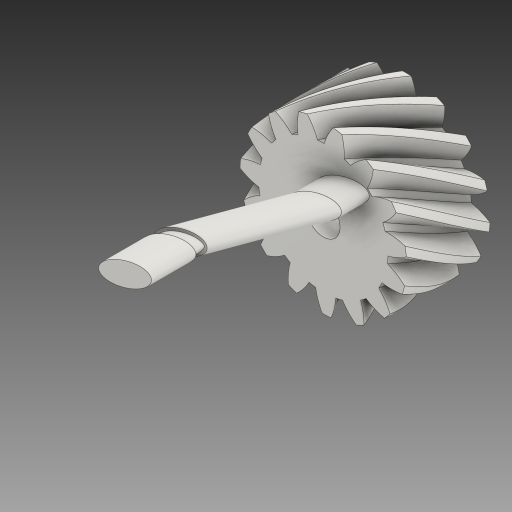
# Autodesk Inventor part: Finger_Profil_V2
Saved by Autodesk Inventor 2024 (Build 280153000, 153)
## iProperties
CustomPartVersion: 1
Created: 2024-03-13
Part Number: Finger_Profil_V2
Material: Steel
Document SubType Name: Modeling
Designer: Faber
Categories: <?xml version="1.0" encoding="UTF-16"?> <MemberInstance><Categories><FamilyTemplate><FamilyTemplateParameter ValueType="xs:double" Id="1" ObjectReferenceKey="da_z" ObjectType="kUserParameterObject"/><FamilyTemplateParameter ValueType="xs:double" Id="2" ObjectReferenceKey="da_b" ObjectType="kUserParameterObject"/><FamilyTemplateParameter ValueType="xs:double" Id="3" ObjectReferenceKey="da_beta" ObjectType="kUserParameterObject"/><FamilyTemplateParameter ValueType="xs:double" Id="4" ObjectReferenceKey="da_da" ObjectType="kUserParameterObject"/><FamilyTemplateParameter ValueType="xs:double" Id="5" ObjectReferenceKey="da_aw" ObjectType="kUserParameterObject"/><FamilyTemplateParameter ValueType="xs:string" Id="6" ObjectReferenceKey="EAIAABAAAACIAQAAAAAAAIAAAAAAAAAA" ObjectType="83910656" SubObjectId="SurfaceGeometry"/></FamilyTemplate><ParamToTemplateMap><ParamToTemplate CategoryParameter="//CategoryParameter[@InternalName='046C89C9-8512-4d59-83FE-43B91F4F132A']" TemplateParameter="1"/><ParamToTemplate CategoryParameter="//CategoryParameter[@InternalName='2552DF32-E462-4b46-AEBF-C6C7768E72AC']" TemplateParameter="2"/><ParamToTemplate CategoryParameter="//CategoryParameter[@InternalName='C9EE641D-15FC-4fae-A226-E94C4372FDD7']" TemplateParameter="3"/><ParamToTemplate><ParamToTemplate CategoryParameter="//CategoryParameter[@InternalName='00B6519A-459B-49c7-AD84-2E56D39A5744']" ConstantValue="0.340699"/></ParamToTemplate><ParamToTemplate><ParamToTemplate CategoryParameter="//CategoryParameter[@InternalName='04B31F0E-C7A6-4894-AA32-9629BEFACF47']" ConstantValue="1.000000"/></ParamToTemplate><ParamToTemplate><ParamToTemplate CategoryParameter="//CategoryParameter[@InternalName='43CBEC2E-7847-49e7-A936-2F7889FCB2D9']" ConstantValue="0.250000"/></ParamToTemplate><ParamToTemplate><ParamToTemplate CategoryParameter="//CategoryParameter[@InternalName='B1EFC894-105D-4ebd-86BF-FA20ED196853']" ConstantValue="0.333500"/></ParamToTemplate><ParamToTemplate><ParamToTemplate CategoryParameter="//CategoryParameter[@InternalName='51175063-3D10-4879-93E8-6246FE8B403D']" ConstantValue="2060000000.000000"/></ParamToTemplate><ParamToTemplate><ParamToTemplate CategoryParameter="//CategoryParameter[@InternalName='A3A52E27-4454-46a9-B0BD-C932399B70AF']" ConstantValue="0.300000"/></ParamToTemplate><ParamToTemplate><ParamToTemplate CategoryParameter="//CategoryParameter[@InternalName='91B76062-C214-41d9-B1B9-14D2AB99603D']" ConstantValue="0.150000"/></ParamToTemplate><ParamToTemplate><ParamToTemplate CategoryParameter="//CategoryParameter[@InternalName='374E806E-8B8A-4dda-A9AA-1039D6500AD2']" ConstantValue="6.666667"/></ParamToTemplate><ParamToTemplate><ParamToTemplate CategoryParameter="//CategoryParameter[@InternalName='2D373A89-B862-43d6-8D0B-0CBF12AB9F6C']" ConstantValue="0.349066"/></ParamToTemplate><ParamToTemplate CategoryParameter="//CategoryParameter[@InternalName='37777632-D6A2-4fac-9D53-DB8ACD95C989']" TemplateParameter="4"/><ParamToTemplate CategoryParameter="//CategoryParameter[@InternalName='FD1017F1-B727-4f7e-9707-0F86F1FF9423']" TemplateParameter="5"/><ParamToTemplate><ParamToTemplate CategoryParameter="//CategoryParameter[@InternalName='9E1B4470-B2D3-4ff1-B813-535BB4CDF51A']" ConstantValue="3520000.000000"/></ParamToTemplate><ParamToTemplate><ParamToTemplate CategoryParameter="//CategoryParameter[@InternalName='F8452263-BFF6-458c-9FB1-07C4B99E95CD']" ConstantValue="11400000.000000"/></ParamToTemplate><ParamToTemplate><ParamToTemplate CategoryParameter="//CategoryParameter[@InternalName='3E3BB259-FD49-497f-8171-6EBC954A3479']" ConstantValue="2.000000"/></ParamToTemplate><ParamToTemplate CategoryParameter="//CategoryParameter[@InternalName='27C3BAF2-7550-4e4b-AE2C-0DB134B7D9B7']" TemplateParameter="6"/></ParamToTemplateMap><Category DisplayName="Gear" InternalName="DC85795E-93AB-48d5-8EEE-5A27447B64BD" Mnemonic="Gear"><CategoryParameter DisplayName="z" InternalName="046C89C9-8512-4d59-83FE-43B91F4F132A" Mnemonic="z"/><CategoryParameter DisplayName="b" InternalName="2552DF32-E462-4b46-AEBF-C6C7768E72AC" Mnemonic="b"/><CategoryParameter DisplayName="||b|" InternalName="C9EE641D-15FC-4fae-A226-E94C4372FDD7" Mnemonic="beta"/><CategoryParameter DisplayName="x" InternalName="00B6519A-459B-49c7-AD84-2E56D39A5744" Mnemonic="x"/><CategoryParameter DisplayName="a*" InternalName="04B31F0E-C7A6-4894-AA32-9629BEFACF47" Mnemonic="a"/><CategoryParameter DisplayName="c*" InternalName="43CBEC2E-7847-49e7-A936-2F7889FCB2D9" Mnemonic="c"/><CategoryParameter DisplayName="r|.f|*" InternalName="B1EFC894-105D-4ebd-86BF-FA20ED196853" Mnemonic="rf"/><CategoryParameter DisplayName="E" InternalName="51175063-3D10-4879-93E8-6246FE8B403D" Mnemonic="E"/><CategoryParameter DisplayName="||m|" InternalName="A3A52E27-4454-46a9-B0BD-C932399B70AF" Mnemonic="mi"/><Category DisplayName="SpurGear" InternalName="26C5A22E-A91E-4dfd-A3B3-23CCAFAE1764" Mnemonic="SpurGear"><CategoryParameter DisplayName="m" InternalName="91B76062-C214-41d9-B1B9-14D2AB99603D" Mnemonic="m"/><CategoryParameter DisplayName="P" InternalName="374E806E-8B8A-4dda-A9AA-1039D6500AD2" Mnemonic="PP"/><CategoryParameter DisplayName="||a|" InternalName="2D373A89-B862-43d6-8D0B-0CBF12AB9F6C" Mnemonic="alpha"/><CategoryParameter DisplayName="d|.a|" InternalName="37777632-D6A2-4fac-9D53-DB8ACD95C989" Mnemonic="da"/><CategoryParameter DisplayName="a|.w|" InternalName="FD1017F1-B727-4f7e-9707-0F86F1FF9423" Mnemonic="aw"/><CategoryParameter DisplayName="||s||.Flim|" InternalName="9E1B4470-B2D3-4ff1-B813-535BB4CDF51A" Mnemonic="sFlim"/><CategoryParameter DisplayName="||s||.Hlim|" InternalName="F8452263-BFF6-458c-9FB1-07C4B99E95CD" Mnemonic="sHlim"/><CategoryParameter DisplayName="type" InternalName="3E3BB259-FD49-497f-8171-6EBC954A3479" Mnemonic="type"/><CategoryParameter DisplayName="PitchDiameter" InternalName="27C3BAF2-7550-4e4b-AE2C-0DB134B7D9B7" Mnemonic="IDS_PITCHDIAM"/></Category></Category></Categories></MemberInstance>
Density: 1 g/cm^3
Appearance: Steel
Author: Faber
## iProperties of the stored document Spur Gear21_3DPrint.ipt
Created: 2024-03-13
Part Number: Spur Gear21_3DPrint
Material: Generic
Document SubType Name: Modeling
Designer: Faber
Density: 1 g/cm^3
Appearance: Default
Author: Faber
Autodesk Inventor part; units mm, degrees
note: some values were not read from the file. Chosen so that the rebuilt part matches the saved one: offset side.
sketch "Sketch1" plane through (0, 0, 0) normal (0, 0, 1) x (1, 0, 0)
  circle A0 centre (0, 0) radius 14.9737
  dimension "d0" = 29.9474
  constraints: 1 centre point
  measures "d0" diameter of A0
extrude "Extrusion1" add sketch "Sketch1" along normal blind 15
ref_plane "Work Plane2" through (0, 0, 7.5) normal (0, 0, 1) x (1, 0, 0)
sketch "Sketch2" plane through (0, 0, 0) normal (0, 0, -1) x (-1, 0, 0)
  circle A0 centre (0, 0) radius 14.9737 projected
  circle A1 centre (0, 0) radius 12.9904
  dimension "d3" = 25.9808
  constraints: 1 centre point, 1 coincident
  measures "d3" diameter of A1
surface extrude "Pitch Diameter" sketch "Sketch2" against normal through all shown no curves A1
ref_plane "Work Plane8" through (0, 0, 0) normal (0.9781476, 0.2079117, 0) x (0, 0, 1)
ref_plane "Work Plane9" through (0, 0, 0) normal (1, 0, 0) x (0, 1, 0)
spur gear teeth "Spur Gear" teeth 15 pitch diameter 25.9808 tip diameter 29.9474 root diameter 23.2529 face width 15 helix angle 30 hand right start plane through (0, 0, 0) normal (0, 0, -1) x (-1, 0, 0)
sketch "Sketch3" plane through (0, 0, 15) normal (0, 0, 1) x (1, 0, 0)
  arc A0 (-4.5796, 10.6865) -> (-5.6716, 10.1492) centre (0, 0) ccw projected
  arc A1 (-4.4271, 14.3043) -> (-4.5796, 10.6865) centre (5.6173, 12.0689) ccw projected
  arc A2 (-1.0532, 11.5786) -> (-2.9077, 14.6887) centre (-10.6807, 7.9457) ccw projected
  arc A3 (0.1629, 11.6253) -> (-1.0532, 11.5786) centre (0, 0) ccw projected
  arc A4 (1.7737, 14.8683) -> (0.1629, 11.6253) centre (10.0405, 8.7407) ccw projected
  arc A5 (3.7473, 11.006) -> (3.3181, 14.6015) centre (-6.5255, 11.603) ccw projected
  arc A6 (4.8772, 10.554) -> (3.7473, 11.006) centre (0, 0) ccw projected
  arc A7 (7.6678, 12.8615) -> (4.8772, 10.554) centre (12.7276, 3.9012) ccw projected
  arc A8 (7.8999, 8.5303) -> (8.9702, 11.9895) centre (-1.242, 13.254) ccw projected
  arc A9 (8.7483, 7.6578) -> (7.8999, 8.5303) centre (0, 0) ccw projected
  arc A10 (12.2361, 8.6307) -> (8.7483, 7.6578) centre (13.214, -1.6129) ccw projected
  arc A11 (10.6865, 4.5796) -> (13.0712, 7.3044) centre (4.2563, 12.6133) ccw projected
  arc A12 (11.1066, 3.4375) -> (10.6865, 4.5796) centre (0, 0) ccw projected
  arc A13 (14.6887, 2.9077) -> (11.1066, 3.4375) centre (11.4156, -6.8481) ccw projected
  arc A14 (11.6253, -0.1629) -> (14.9122, 1.3564) centre (9.0186, 9.7917) ccw projected
  arc A15 (11.5446, -1.3772) -> (11.6253, -0.1629) centre (0, 0) ccw projected
  arc A16 (14.6015, -3.3181) -> (11.5446, -1.3772) centre (7.6433, -10.8992) ccw projected
  arc A17 (10.554, -4.8772) -> (14.1746, -4.8262) centre (12.2215, 5.2769) ccw projected
  arc A18 (9.9863, -5.9537) -> (10.554, -4.8772) centre (0, 0) ccw projected
  arc A19 (11.9895, -8.9702) -> (9.9863, -5.9537) centre (2.5494, -13.0657) ccw projected
  arc A20 (7.6578, -8.7483) -> (10.9862, -10.1743) centre (13.3112, -0.1502) ccw projected
  arc A21 (6.7014, -9.5008) -> (7.6578, -8.7483) centre (0, 0) ccw projected
  arc A22 (7.3044, -13.0712) -> (6.7014, -9.5008) centre (-2.9853, -12.973) ccw projected
  arc A23 (3.4375, -11.1066) -> (5.8981, -13.7632) centre (12.0993, -5.5514) ccw projected
  arc A24 (2.2577, -11.4051) -> (3.4375, -11.1066) centre (0, 0) ccw projected
  arc A25 (1.3564, -14.9122) -> (2.2577, -11.4051) centre (-8.0038, -10.6372) ccw projected
  arc A26 (-1.3772, -11.5446) -> (-0.2098, -14.9723) centre (8.7953, -9.9927) ccw projected
  arc A27 (-2.5764, -11.3374) -> (-1.3772, -11.5446) centre (0, 0) ccw projected
  arc A28 (-4.8262, -14.1746) -> (-2.5764, -11.3374) centre (-11.6384, -6.4622) ccw projected
  arc A29 (-5.9537, -9.9863) -> (-6.2814, -13.5925) centre (3.9705, -12.7062) ccw projected
  arc A30 (-6.965, -9.3093) -> (-5.9537, -9.9863) centre (0, 0) ccw projected
  arc A31 (-10.1743, -10.9862) -> (-6.965, -9.3093) centre (-13.2606, -1.1697) ccw projected
  arc A32 (-9.5008, -6.7014) -> (-11.2669, -9.8625) centre (-1.5408, -13.2226) ccw projected
  arc A33 (-10.1492, -5.6716) -> (-9.5008, -6.7014) centre (0, 0) ccw projected
  arc A34 (-13.7632, -5.8981) -> (-10.1492, -5.6716) centre (-12.5899, 4.325) ccw projected
  arc A35 (-11.4051, -2.2577) -> (-14.3043, -4.4271) centre (-6.7857, -11.4528) ccw projected
  arc A36 (-11.5786, -1.0532) -> (-11.4051, -2.2577) centre (0, 0) ccw projected
  arc A37 (-14.9723, 0.2098) -> (-11.5786, -1.0532) centre (-9.7423, 9.0718) ccw projected
  arc A38 (-11.3374, 2.5764) -> (-14.8683, 1.7737) centre (-10.8573, -7.7026) ccw projected
  arc A39 (-11.006, 3.7473) -> (-11.3374, 2.5764) centre (0, 0) ccw projected
  arc A40 (-13.5925, 6.2814) -> (-11.006, 3.7473) centre (-5.2102, 12.2501) ccw projected
  arc A41 (-5.6716, 10.1492) -> (-8.6307, 12.2361) centre (-12.9891, 2.9145) ccw projected
  circle A42 centre (0, 0) radius 3
  arc A43 (-2.9077, 14.6887) -> (-4.4271, 14.3043) centre (0, 0) ccw projected
  arc A44 (3.3181, 14.6015) -> (1.7737, 14.8683) centre (0, 0) ccw projected
  arc A45 (8.9702, 11.9895) -> (7.6678, 12.8615) centre (0, 0) ccw projected
  arc A46 (13.0712, 7.3044) -> (12.2361, 8.6307) centre (0, 0) ccw projected
  arc A47 (14.9122, 1.3564) -> (14.6887, 2.9077) centre (0, 0) ccw projected
  arc A48 (14.1746, -4.8262) -> (14.6015, -3.3181) centre (0, 0) ccw projected
  arc A49 (10.9862, -10.1743) -> (11.9895, -8.9702) centre (0, 0) ccw projected
  arc A50 (5.8981, -13.7632) -> (7.3044, -13.0712) centre (0, 0) ccw projected
  arc A51 (-0.2098, -14.9723) -> (1.3564, -14.9122) centre (0, 0) ccw projected
  arc A52 (-6.2814, -13.5925) -> (-4.8262, -14.1746) centre (0, 0) ccw projected
  arc A53 (-11.2669, -9.8625) -> (-10.1743, -10.9862) centre (0, 0) ccw projected
  arc A54 (-14.3043, -4.4271) -> (-13.7632, -5.8981) centre (0, 0) ccw projected
  arc A55 (-14.8683, 1.7737) -> (-14.9723, 0.2098) centre (0, 0) ccw projected
  arc A56 (-8.6307, 12.2361) -> (-9.8625, 11.2669) centre (0, 0) ccw projected
  arc A57 (-12.8615, 7.6678) -> (-13.5925, 6.2814) centre (0, 0) ccw projected
  dimension "d49" = 6
  constraints: 1 centre point, 1 coincident, 3 other
  measures "d49" diameter of A42
extrude "Axes" cut sketch "Sketch3" against normal through all
sketch "Sketch4" plane through (0, 0, 15) normal (0, 0, 1) x (1, 0, 0)
  circle A0 centre (0, 0) radius 3 projected
  arc A1 (-4.5796, 10.6865) -> (-5.6716, 10.1492) centre (0, 0) ccw projected
  arc A2 (-4.4271, 14.3043) -> (-4.5796, 10.6865) centre (5.6173, 12.0689) ccw projected
  arc A3 (-1.0532, 11.5786) -> (-2.9077, 14.6887) centre (-10.6807, 7.9457) ccw projected
  arc A4 (0.1629, 11.6253) -> (-1.0532, 11.5786) centre (0, 0) ccw projected
  arc A5 (1.7737, 14.8683) -> (0.1629, 11.6253) centre (10.0405, 8.7407) ccw projected
  arc A6 (3.7473, 11.006) -> (3.3181, 14.6015) centre (-6.5255, 11.603) ccw projected
  arc A7 (4.8772, 10.554) -> (3.7473, 11.006) centre (0, 0) ccw projected
  arc A8 (7.6678, 12.8615) -> (4.8772, 10.554) centre (12.7276, 3.9012) ccw projected
  arc A9 (7.8999, 8.5303) -> (8.9702, 11.9895) centre (-1.242, 13.254) ccw projected
  arc A10 (8.7483, 7.6578) -> (7.8999, 8.5303) centre (0, 0) ccw projected
  arc A11 (12.2361, 8.6307) -> (8.7483, 7.6578) centre (13.214, -1.6129) ccw projected
  arc A12 (10.6865, 4.5796) -> (13.0712, 7.3044) centre (4.2563, 12.6133) ccw projected
  arc A13 (11.1066, 3.4375) -> (10.6865, 4.5796) centre (0, 0) ccw projected
  arc A14 (14.6887, 2.9077) -> (11.1066, 3.4375) centre (11.4156, -6.8481) ccw projected
  arc A15 (11.6253, -0.1629) -> (14.9122, 1.3564) centre (9.0186, 9.7917) ccw projected
  arc A16 (11.5446, -1.3772) -> (11.6253, -0.1629) centre (0, 0) ccw projected
  arc A17 (14.6015, -3.3181) -> (11.5446, -1.3772) centre (7.6433, -10.8992) ccw projected
  arc A18 (10.554, -4.8772) -> (14.1746, -4.8262) centre (12.2215, 5.2769) ccw projected
  arc A19 (9.9863, -5.9537) -> (10.554, -4.8772) centre (0, 0) ccw projected
  arc A20 (11.9895, -8.9702) -> (9.9863, -5.9537) centre (2.5494, -13.0657) ccw projected
  arc A21 (7.6578, -8.7483) -> (10.9862, -10.1743) centre (13.3112, -0.1502) ccw projected
  arc A22 (6.7014, -9.5008) -> (7.6578, -8.7483) centre (0, 0) ccw projected
  arc A23 (7.3044, -13.0712) -> (6.7014, -9.5008) centre (-2.9853, -12.973) ccw projected
  arc A24 (3.4375, -11.1066) -> (5.8981, -13.7632) centre (12.0993, -5.5514) ccw projected
  arc A25 (2.2577, -11.4051) -> (3.4375, -11.1066) centre (0, 0) ccw projected
  arc A26 (1.3564, -14.9122) -> (2.2577, -11.4051) centre (-8.0038, -10.6372) ccw projected
  arc A27 (-1.3772, -11.5446) -> (-0.2098, -14.9723) centre (8.7953, -9.9927) ccw projected
  arc A28 (-2.5764, -11.3374) -> (-1.3772, -11.5446) centre (0, 0) ccw projected
  arc A29 (-4.8262, -14.1746) -> (-2.5764, -11.3374) centre (-11.6384, -6.4622) ccw projected
  arc A30 (-5.9537, -9.9863) -> (-6.2814, -13.5925) centre (3.9705, -12.7062) ccw projected
  arc A31 (-6.965, -9.3093) -> (-5.9537, -9.9863) centre (0, 0) ccw projected
  arc A32 (-10.1743, -10.9862) -> (-6.965, -9.3093) centre (-13.2606, -1.1697) ccw projected
  arc A33 (-9.5008, -6.7014) -> (-11.2669, -9.8625) centre (-1.5408, -13.2226) ccw projected
  arc A34 (-10.1492, -5.6716) -> (-9.5008, -6.7014) centre (0, 0) ccw projected
  arc A35 (-13.7632, -5.8981) -> (-10.1492, -5.6716) centre (-12.5899, 4.325) ccw projected
  arc A36 (-11.4051, -2.2577) -> (-14.3043, -4.4271) centre (-6.7857, -11.4528) ccw projected
  arc A37 (-11.5786, -1.0532) -> (-11.4051, -2.2577) centre (0, 0) ccw projected
  arc A38 (-14.9723, 0.2098) -> (-11.5786, -1.0532) centre (-9.7423, 9.0718) ccw projected
  arc A39 (-11.3374, 2.5764) -> (-14.8683, 1.7737) centre (-10.8573, -7.7026) ccw projected
  arc A40 (-11.006, 3.7473) -> (-11.3374, 2.5764) centre (0, 0) ccw projected
  arc A41 (-13.5925, 6.2814) -> (-11.006, 3.7473) centre (-5.2102, 12.2501) ccw projected
  arc A42 (-5.6716, 10.1492) -> (-8.6307, 12.2361) centre (-12.9891, 2.9145) ccw projected
  ellipse E0 centre (3.5, 6.0622) end of major axis (8.1985, 7.7723) minor radius 2
  line L0 (0, 0) -> (-9.9607, 0) construction
  circle A43 centre (0, 0) radius 7 construction
  line L1 (3.5, 6.0622) -> (0, 0) construction
  arc A44 (-2.9077, 14.6887) -> (-4.4271, 14.3043) centre (0, 0) ccw projected
  arc A45 (3.3181, 14.6015) -> (1.7737, 14.8683) centre (0, 0) ccw projected
  arc A46 (8.9702, 11.9895) -> (7.6678, 12.8615) centre (0, 0) ccw projected
  arc A47 (13.0712, 7.3044) -> (12.2361, 8.6307) centre (0, 0) ccw projected
  arc A48 (14.9122, 1.3564) -> (14.6887, 2.9077) centre (0, 0) ccw projected
  arc A49 (14.1746, -4.8262) -> (14.6015, -3.3181) centre (0, 0) ccw projected
  arc A50 (10.9862, -10.1743) -> (11.9895, -8.9702) centre (0, 0) ccw projected
  arc A51 (5.8981, -13.7632) -> (7.3044, -13.0712) centre (0, 0) ccw projected
  arc A52 (-0.2098, -14.9723) -> (1.3564, -14.9122) centre (0, 0) ccw projected
  arc A53 (-6.2814, -13.5925) -> (-4.8262, -14.1746) centre (0, 0) ccw projected
  arc A54 (-11.2669, -9.8625) -> (-10.1743, -10.9862) centre (0, 0) ccw projected
  arc A55 (-14.3043, -4.4271) -> (-13.7632, -5.8981) centre (0, 0) ccw projected
  arc A56 (-14.8683, 1.7737) -> (-14.9723, 0.2098) centre (0, 0) ccw projected
  arc A57 (-8.6307, 12.2361) -> (-9.8625, 11.2669) centre (0, 0) ccw projected
  arc A58 (-12.8615, 7.6678) -> (-13.5925, 6.2814) centre (0, 0) ccw projected
  circle A59 centre (0, 0) radius 23 construction
  line L2 (15, 38) -> (-15, 38) construction
  line L3 (-15, 38) -> (-15, 8) construction
  line L4 (-15, 8) -> (15, 8) construction
  line L5 (15, 8) -> (15, 38) construction
  line L6 (15, 38) -> (-15, 8) construction
  line L7 (-15, 38) -> (15, 8) construction
  circle A60 centre (0, 23) radius 10 construction
  line L8 (-1.1985, 4.3521) -> (8.1985, 7.7723) construction
  line L9 (-1.1985, 4.3521) -> (0, 0) construction
  line L10 (0, 0) -> (7.091, 5.7594) construction
  point P0 (0, 0)
  point P1 (5.2815, 4.6433)
  dimension "d60" = 2
  dimension "d61" = 5
  dimension "d90" = 14
  dimension "d150" = 46
  dimension "d151" = 30
  dimension "d152" = 30
  dimension "d153" = 20
  dimension "d154" = 120
  dimension "d155" = -20
  dimension "d158" = 66.312
  constraints: 22 end point, 4 coincident, 2 horizontal, 2 midpoint, 2 parallel, 2 vertical alignment, 1 centre point, 1 perpendicular, 21 other
  measures "d151" distance of L2.start L2.end
  measures "d152" distance of L4.end L2.start
  measures "d153" diameter of A60
  measures "d154" angle of L0 L1
  measures "d155" angle of L0 L8
  measures "d158" angle of L9 L10
extrude "Finger_Base" add sketch "Sketch4" along normal blind 5 contours E0
sketch "Sketch6" plane through (0, 0, 20) normal (0, 0, 1) x (1, 0, 0)
  ellipse E0 centre (3.5, 6.0622) end of major axis (8.1985, 7.7723) minor radius 2 projected
  line L0 (-0.4355, 6.0622) -> (7.4355, 6.0622) construction
  point P0 (0, 0)
  constraints: 2 end point, 1 horizontal, 1 midpoint, 3 other
ref_plane "Work Plane11" through (-0.4355, 6.0622, 20) normal (0, -0.9659258, 0.258819) x (1, 0, 0)
sketch "Sketch7" plane through (-0.4355, 6.0622, 20) normal (0, -0.9659258, 0.258819) x (1, 0, 0)
  line L0 (0, 0) -> (7.871, 0) construction
  line L1 (3.9355, 0) -> (3.9355, 25)
  point P0 (0.4355, -20.8875)
  dimension "d76" = 25
  constraints: 2 end point, 1 perpendicular, 1 vertical
  measures "d76" distance of L1.start L1.end
sweep "Finger_Body" add profiles "Sketch6" path "Sketch7"
sketch "Sketch8" plane through (3.5, 12.5327, 44.1481) normal (0, 0, 1) x (0.9396926, 0.3420201, 0)
  ellipse E0 centre (0, 0) end of major axis (-5, 0) minor radius 2 projected
  point P0 (-7.5753, -10.5798)
  constraints: 1 other
extrude "Finger_Tip" add sketch "Sketch8" along normal blind 10
ref_plane "Rib_Offset" through (3.5, 12.5327, 46.1481) normal (0, 0, 1) x (0.9396926, 0.3420201, 0)
sketch "Sketch9" plane through (3.5, 12.5327, 46.1481) normal (0, 0, 1) x (0.9396926, 0.3420201, 0)
  ellipse E0 centre (0, 0) end of major axis (-5, 0) minor radius 2 projected
  spline S0 degree 5 poles (-4.5, 0) (-4.5007, -0.096) (-4.4576, -0.189) (-4.4038, -0.2671) (-4.198, -0.5027) (-3.9339, -0.675) (-3.7457, -0.7795) (-3.2634, -1.0024) (-2.7562, -1.1611) (-2.4507, -1.2391) (-1.7817, -1.3778) (-1.1029, -1.4577) (-0.7358, -1.4859) (0, -1.5141) (0.7358, -1.4859) (1.1029, -1.4576) (1.7817, -1.3779) (2.4506, -1.239) (2.7563, -1.1612) (3.2633, -1.0022) (3.7458, -0.7797) (3.9338, -0.6745) (4.1982, -0.5032) (4.4036, -0.2665) (4.4583, -0.1904) (4.542, 0) (4.4583, 0.1904) (4.4036, 0.2665) (4.1982, 0.5032) (3.9338, 0.6745) (3.7458, 0.7797) (3.2633, 1.0022) (2.7563, 1.1612) (2.4506, 1.239) (1.7817, 1.3779) (1.1029, 1.4576) (0.7358, 1.4859) (0, 1.5141) (-0.7358, 1.4859) (-1.1029, 1.4577) (-1.7817, 1.3778) (-2.4507, 1.2391) (-2.7562, 1.1611) (-3.2634, 1.0024) (-3.7457, 0.7795) (-3.9339, 0.675) (-4.198, 0.5027) (-4.4038, 0.2671) (-4.4576, 0.189) (-4.5007, 0.096) (-4.5, 0) knots 0 0 0 0 0 0 0.024023 0.024023 0.024023 0.078224 0.078224 0.078224 0.157431 0.157431 0.157431 0.25 0.25 0.25 0.342566 0.342566 0.342566 0.42178 0.42178 0.42178 0.47598 0.47598 0.47598 0.5 0.5 0.5 0.52402 0.52402 0.52402 0.57822 0.57822 0.57822 0.657434 0.657434 0.657434 0.75 0.75 0.75 0.842569 0.842569 0.842569 0.921776 0.921776 0.921776 0.975977 0.975977 0.975977 1 1 1 1 1 1
  point P0 (-7.5753, -10.5798)
  dimension "d82" = 0.5
  constraints: 1 other
extrude "Tip_Rib" cut sketch "Sketch9" against normal blind 2
sketch "Sketch16" plane through (3.5, 12.5327, 54.1481) normal (0, 0, 1) x (0.9396926, 0.3420201, 0)
  ellipse E0 centre (0, 0) end of major axis (-5, 0) minor radius 2 projected
  circle A0 centre (-7.5753, -10.5798) radius 16.6589 construction
  line L0 (-7.5753, -10.5798) -> (4.6932, 0.6898) construction
  line L1 (9.2562, -8.1925) -> (19.5168, 19.9982) construction
  line L2 (9.2562, -8.1925) -> (8.9987, -8.9) construction
  line L3 (-7.5753, -10.5798) -> (8.9987, -8.9) construction
  dimension "d157" = 36.783
  constraints: 6 end point, 2 point on circle, 1 centre point, 1 coincident, 1 collinear, 3 other
  measures "d157" angle of L0 L3
equation "\"d0\" = da_da"
equation "\"d1\" = da_b"
equation "\"d3\" = da_d"
equation "\"d16\" = da_aw"
equation "\"d43\" = da_aw"
equation "\"d46\" = da_aw"
equation "\"da_da\" = 29.947441"
equation "\"da_b\" = 15"
equation "\"da_d\" = 25.980762"
equation "\"da_aw\" = 23"
body "Solid1"
body "Srf1"
